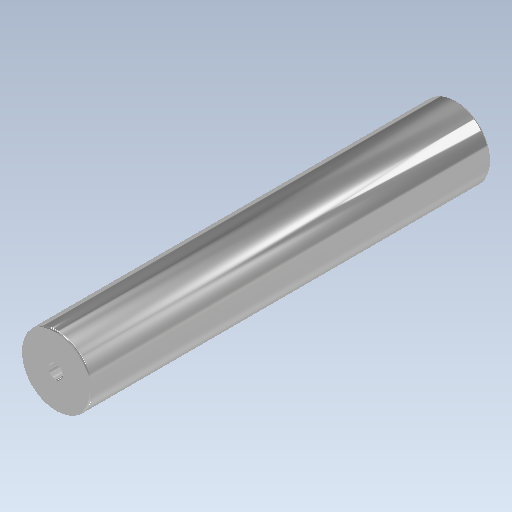
# Autodesk Inventor part: ADSK-MH-10022
Saved by Autodesk Inventor 2021.1 (Build 251245010, 245A)
## iProperties
Created: 2008-03-10
Part Number: ADSK-MH-10022
Document SubType Name: Modeling
Designer: R.O'mahony
Density: 7.86 g/cm^3
Mass: 329.975 g
Surface Area: 331.968 cm^2
Volume: 329.975 cm^3
Material: Steel, Mild
Appearance: Chrome - Polished
Description: Roller Shaft
Engineer: Demir Ali
Checked By: Demir Ali
Company: Autodesk Ltd
Author: R.O'mahony
Keywords: Roller Conveyor
Revision Number: A
Autodesk Inventor part; units mm, degrees
ref_plane "YZ Plane" through (0, 0, 0) normal (1, 0, 0) x (0, 1, 0)
ref_plane "XZ Plane" through (0, 0, 0) normal (0, 1, 0) x (-1, 0, 0)
ref_plane "XY Plane" through (0, 0, 0) normal (0, 0, 1) x (1, 0, 0)
sketch "Sketch1" plane through (0, 0, 0) normal (0, 0, 1) x (1, 0, 0)
  circle A0 centre (0, 0) radius 35
  circle A1 centre (0, 0) radius 7.2917
  dimension "d0" = 70
  constraints: 2 centre point, 1 coincident
  measures "d0" diameter of A0
extrude "Extrusion1" add sketch "Sketch1" against normal blind 400
fillet "Fillet1" radius 2 2 edges at (-35, 0, 0) (-35, 0, -400)
body "Solid1"
